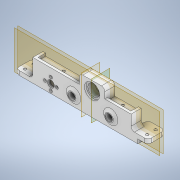
# Autodesk Inventor part: MotorBracketv2
Saved by Autodesk Inventor 2022 (Build 260153000, 153)
## iProperties
Created: 2022-01-31
Part Number: MotorBracketv2
Material: ABS プラスチック
Document SubType Name: Modeling
Designer: shiokaze
Density: 1.06 g/cm^3
Appearance: 滑らか - 白
Mass: 5.74152 g
Surface Area: 41.0545 cm^2
Volume: 5.41653 cm^3
Author: shiokaze
Autodesk Inventor part; units mm, degrees
ref_plane "YZ Plane" through (0, 0, 0) normal (1, 0, 0) x (0, 1, 0)
ref_plane "XZ Plane" through (0, 0, 0) normal (0, 1, 0) x (-1, 0, 0)
ref_plane "XY Plane" through (0, 0, 0) normal (0, 0, 1) x (1, 0, 0)
sketch "スケッチ2" plane through (0, 0, 0) normal (0, 0, 1) x (1, 0, 0)
  line L0 (-46.5, 9.45) -> (31.5, 9.45)
  line L1 (31.5, 9.45) -> (31.5, -9.45)
  line L2 (31.5, -9.45) -> (-46.5, -9.45)
  line L3 (-46.5, -9.45) -> (-46.5, 9.45)
  line L4 (-46.5, 9.45) -> (31.5, -9.45)
  line L5 (31.5, 9.45) -> (-46.5, -9.45)
  line L6 (-46.5, 9.45) -> (-9, 9.45)
  line L7 (-9, 9.45) -> (-9, -6.95)
  line L8 (-9, -6.95) -> (-46.5, -6.95)
  line L9 (-46.5, -6.95) -> (-46.5, 9.45)
  line L10 (31.5, 9.45) -> (6, 9.45)
  line L11 (6, 9.45) -> (6, -4.45)
  line L12 (6, -4.45) -> (31.5, -4.45)
  line L13 (31.5, -4.45) -> (31.5, 9.45)
  line L14 (-36.1825, -6.95) -> (-36.5, -6.95)
  line L15 (-36.5, -6.95) -> (-36.5, 3.75)
  line L16 (-36.5, 3.75) -> (-9, 3.75)
  line L17 (-9, 3.75) -> (-9, -0.3635)
  line L18 (6, -4.45) -> (21.5, -4.45)
  line L19 (21.5, -4.45) -> (21.5, 3.75)
  line L20 (21.5, 3.75) -> (6, 3.75)
  line L21 (6, 3.75) -> (6, -4.45)
  line L22 (31.5, -9.45) -> (25.5, -9.45)
  line L23 (25.5, -9.45) -> (25.5, -6.95)
  line L24 (25.5, -6.95) -> (31.5, -6.95)
  line L25 (31.5, -6.95) -> (31.5, -9.45)
  line L26 (-7.5, 0) -> (0, 0)
  point P0 (-7.5, 0)
  point P1 (6, 3.75)
  point P2 (6, 9.45)
  point P3 (-9, 9.45)
  point P4 (-9, 3.75)
  point P5 (-36.5, -6.95)
  point P6 (25.5, -9.45)
  point P7 (31.5, -6.95)
  point P8 (31.5, -4.45)
  dimension "d0" = 78
  dimension "d1" = 18.9
  dimension "d15" = 37.5
  dimension "d16" = 2.5
  dimension "d17" = 25.5
  dimension "d18" = 6
  dimension "d19" = 2.5
  dimension "d20" = 10
  dimension "d21" = 10
  dimension "d26" = 7.5
  dimension "d188" = 10.7
  dimension "d241" = 5
  constraints: 54 end point, 12 parallel, 7 horizontal, 6 perpendicular, 3 collinear, 2 midpoint, 2 point on line, 1 coincident
  measures "d0" distance of L0.start L0.end
  measures "d1" distance of L0.end L1.end
  measures "d15" distance of L7.end L8.end
  measures "d16" distance between parallel lines of L2 L8
  measures "d17" distance of L12.end L11.end
  measures "d18" distance of L23.end L24.end
  measures "d19" distance of L22.end L23.end
  measures "d20" distance between parallel lines of L1 L19
  measures "d21" distance between parallel lines of L3 L15
  measures "d26" distance of L26.start L26.end
  measures "d188" distance between parallel lines of L16 L8
  measures "d241" distance between parallel lines of L18 L2
extrude "押し出し1" add sketch "スケッチ2" along normal blind 6 contours L0 L11 L5 L4 L7 | L8 L5 L3 | L16 L7 L4 | L4 L7 L5 L8 L15 L16 | L5 L8 L7 L4 L11 L12 L23 L2 | L4 L5 L7 | L20 L5 L11 | L5 L7 L8 | L5 L11 L4 | L1 L24 L23 L4 L12 | L20 L19 L12 L4 L11 L5 | L4 L12 L11
sketch "スケッチ8" plane through (0, 0, 6) normal (0, 0, 1) x (1, 0, 0)
  circle A0 centre (-1.5, 4.0146) radius 3.75 construction
  circle A1 centre (9.5, -3.55) radius 9.6 construction
  circle A2 centre (-12.5, -3.55) radius 9.6 construction
  circle A3 centre (-25.8196, -4.45) radius 3.75 construction
  line L0 (-46.5, -9.45) -> (25.5, -9.45) construction
  circle A4 centre (-12.5, -3.55) radius 10
  circle A5 centre (9.5, -3.55) radius 10
  line L1 (-2.5, -3.55) -> (-0.5, -3.55)
  line L2 (-12.5, -3.55) -> (-1.5, 4.0146) construction
  line L3 (-1.5, 4.0146) -> (9.5, -3.55) construction
  line L4 (-25.8196, -4.45) -> (-12.5, -3.55) construction
  line L5 (-46.5, -9.45) -> (25.5, -9.45) projected
  line L6 (-46.5, -9.45) -> (25.5, -9.45)
  line L7 (25.5, -9.45) -> (25.5, -11.05)
  line L8 (25.5, -11.05) -> (-46.5, -11.05) construction
  line L9 (-46.5, -11.05) -> (-46.5, -9.45)
  line L10 (-46.5, -11.05) -> (25.5, -11.05)
  line L11 (25.5, -11.05) -> (25.5, -13.55)
  line L12 (25.5, -13.55) -> (-46.5, -13.55) construction
  line L13 (-46.5, -13.55) -> (-46.5, -11.05)
  line L14 (25.5, -9.45) -> (25.5, -6.95) projected
  line L15 (6, 9.45) -> (-9, 9.45) projected
  circle A6 centre (-25.8196, -4.45) radius 5
  point P0 (0, 0)
  point P1 (-1.5, 9.45)
  dimension "d123" = 20
  dimension "d124" = 20
  dimension "d29" = 7.5
  dimension "d30" = 19.2
  dimension "d31" = 19.2
  dimension "d32" = 7.5
  dimension "d132" = 2
  dimension "d147" = 1.6
  dimension "d148" = 2.5
  dimension "d164" = 10
  constraints: 24 end point, 7 coincident, 5 centre point, 4 horizontal, 4 parallel, 2 collinear, 2 equal length, 2 horizontal alignment, 2 perpendicular, 2 point on line, 2 tangent, 1 midpoint, 1 vertical alignment, 4 other
  measures "d29" diameter of A0
  measures "d30" diameter of A2
  measures "d31" diameter of A1
  measures "d32" diameter of A3
  measures "d132" distance of L1.start L1.end
  measures "d147" distance of L6.end L7.end
  measures "d148" distance of L10.end L11.end
  measures "d164" diameter of A6
hole "穴1" at (-12.5, -3.55, 6) at (9.5, -3.55, 6) at (-1.5, 4.0146, 6) at (-25.8196, -4.45, 6) direction (0, 0, -1) diameter 0.1 end through all
sketch "スケッチ22" plane through (0, 0, 6) normal (0, 0, 1) x (1, 0, 0)
  circle A0 centre (9.5, -3.55) radius 0.05 projected
  circle A1 centre (-12.5, -3.55) radius 0.05 projected
  circle A2 centre (-25.8196, -4.45) radius 0.05 projected
  point P0 (0, 0)
  constraints: 3 coincident
hole "穴8" at (-12.5, -3.55, 6) at (9.5, -3.55, 6) direction (0, 0, -1) diameter 4 end through all
sketch "スケッチ23" plane through (0, 0, 6) normal (0, 0, 1) x (1, 0, 0)
  circle A0 centre (-1.5, 4.0146) radius 0.05 projected
  point P0 (0, 0)
  constraints: 1 coincident
hole "穴9" at (-1.5, 4.0146, 6) direction (0, 0, -1) diameter 7 end through all
sketch "スケッチ27" plane through (0, 0, 6) normal (0, 0, 1) x (1, 0, 0)
  circle A0 centre (-25.8196, -4.45) radius 0.05 projected
  point P0 (0, 0)
  constraints: 1 coincident
hole "穴10" at (-25.8196, -4.45, 6) direction (0, 0, -1) diameter 10 end through all
sketch "スケッチ28" plane through (0, 0, 6) normal (0, 0, 1) x (1, 0, 0)
  circle A0 centre (-25.8196, -4.45) radius 5 projected
  circle A1 centre (-25.8196, -4.45) radius 2
  point P0 (0, 0)
  point P1 (-25.8196, -9.45)
  dimension "d173" = 4
  constraints: 1 centre point, 1 coincident, 1 vertical alignment
  measures "d173" diameter of A1
extrude "押し出し8" add sketch "スケッチ28" against normal blind 1.5
sketch "スケッチ29" plane through (-25.8196, -4.45, 4.5) normal (0, 0, -1) x (-1, 0, 0)
  circle A0 centre (0, 0) radius 2 projected
  point P0 (-25.8196, 4.45)
  point P1 (-3.5, 0)
  point P2 (0, 3.5)
  point P3 (3.5, 0)
  point P4 (0, -3.5)
  dimension "d176" = 3.5
  dimension "d179" = 360
  constraints: 1 coincident, 1 horizontal alignment, 5 other
  measures "d176" distance of point (0, 0) point (-3.5, 0)
hole "穴11" at (-22.3196, -4.45, 4.5) at (-25.8196, -4.45, 4.5) at (-25.8196, -0.95, 4.5) at (-29.3196, -4.45, 4.5) at (-25.8196, -7.95, 4.5) direction (0, 0, 1) diameter 1.8 end through all
sketch "スケッチ30" plane through (0, 0, 0) normal (0, 0, -1) x (-1, 0, 0)
  circle A0 centre (1.5, 4.0146) radius 3.5 projected
  circle A1 centre (1.5, 4.0146) radius 4.5
  point P0 (0, 0)
  dimension "d189" = 9
  constraints: 1 centre point, 1 coincident
  measures "d189" diameter of A1
extrude "押し出し9" cut sketch "スケッチ30" against normal blind 1
sketch "スケッチ31" plane through (-46.5, -9.45, 6) normal (0, -1, 0) x (1, 0, 0)
  line L0 (49.5, -7.5) -> (40.5, -7.5)
  line L1 (40.5, -7.5) -> (40.5, -2.5)
  line L2 (40.5, -2.5) -> (49.5, -2.5)
  line L3 (49.5, -2.5) -> (49.5, -7.5)
  line L4 (49.5, -6) -> (40.5, -6) projected
  line L5 (49.5, -5) -> (40.5, -5) projected
  line L6 (49.5, -6) -> (40.5, -6) projected
  line L7 (0, 0) -> (72, 0) projected
  line L8 (55, -1.6369) -> (35, -1.6369)
  line L9 (35, -1.6369) -> (35, -10)
  line L10 (35, -10) -> (55, -10)
  line L11 (55, -10) -> (55, -1.6369)
  point P0 (46.5, -6)
  point P1 (45, -10)
  point P2 (45, -7.5)
  dimension "d192" = 5
  dimension "d193" = 7.5
  dimension "d194" = 10
  dimension "d195" = 20
  constraints: 16 end point, 4 midpoint, 4 parallel, 2 horizontal, 2 perpendicular, 1 vertical alignment
  measures "d192" distance between parallel lines of L0 L2
  measures "d193" distance between parallel lines of L0 L7
  measures "d194" distance between parallel lines of L10 L7
  measures "d195" distance of L9.end L10.end
extrude "押し出し10" add sketch "スケッチ31" against normal blind 1.5
sketch "スケッチ32" plane through (-46.5, -9.45, 6) normal (0, -1, 0) x (1, 0, 0)
  line L0 (52.5, -7.5) -> (37.5, -7.5)
  line L1 (52.5, -7.5) -> (37.5, -7.5)
  line L2 (37.5, -7.5) -> (37.5, -2.5)
  line L3 (37.5, -2.5) -> (52.5, -2.5)
  line L4 (52.5, -2.5) -> (52.5, -7.5)
  line L5 (37.5, -7.5) -> (37.5, -6)
  line L6 (41.5, -5) -> (48.5, -5) projected
  line L7 (0, 0) -> (72, 0) projected
  point P0 (45, -2.5)
  point P1 (45, -5)
  dimension "d198" = 5
  dimension "d204" = 15
  dimension "d205" = 2.5
  constraints: 12 end point, 2 midpoint, 2 parallel, 1 collinear, 1 horizontal, 1 perpendicular, 1 vertical alignment
  measures "d198" distance of L1.end L2.end
  measures "d204" distance between parallel lines of L4 L2
  measures "d205" distance between parallel lines of L3 L7
extrude "押し出し11" add sketch "スケッチ32" along normal blind 1.6
sketch "スケッチ33" plane through (-46.5, -9.45, 6) normal (0, 1, 0) x (1, 0, 0)
  line L0 (52.5, 2.5) -> (37.5, 2.5) projected
  line L1 (37.5, 2.5) -> (37.5, 7.5) projected
  line L2 (37.5, 7.5) -> (52.5, 7.5) projected
  line L3 (52.5, 7.5) -> (52.5, 2.5) projected
extrude "押し出し12" add sketch "スケッチ33" along normal up to surface (1.5 mm away)
fillet "フィレット14" radius 2 4 edges at (6, -10.25, -1.5) (6, -10.25, 3.5) (-9, -10.25, -1.5) (-9, -10.25, 3.5)
sketch "スケッチ34" plane through (0, 0, 0) normal (0, 0, -1) x (-1, 0, 0)
  line L0 (-31.5, -4.45) -> (-21.5, -4.45) projected
  line L1 (-31.5, -6.95) -> (-31.5, -4.45) projected
  line L2 (-25.5, -6.95) -> (-31.5, -6.95) projected
  line L3 (-8.5, -9.45) -> (-25.5, -9.45) projected
  line L4 (-25.5, -9.45) -> (-25.5, -6.95) projected
  line L5 (-21.5, -4.45) -> (-21.5, 3.75) projected
  line L6 (36.5, -6.95) -> (46.5, -6.95) projected
  line L7 (36.5, 3.75) -> (36.5, -6.95) projected
  line L8 (46.5, -9.45) -> (25.8196, -9.45) projected
  line L9 (46.5, -6.95) -> (46.5, -9.45) projected
  line L10 (-31.5, -4.45) -> (-21.5, -4.45)
  line L11 (-21.5, -4.45) -> (-21.5, -6.95)
  line L12 (-21.5, -6.95) -> (-31.5, -6.95)
  line L13 (-31.5, -6.95) -> (-31.5, -4.45)
  line L14 (46.5, -9.45) -> (-25.5, -9.45) projected
  line L15 (-21.5, -9.45) -> (-25.5, -9.45)
  line L16 (-25.5, -9.45) -> (-25.5, -6.95)
  line L17 (-25.5, -6.95) -> (-21.5, -6.95)
  line L18 (-21.5, -6.95) -> (-21.5, -9.45)
  line L19 (36.5, -6.95) -> (46.5, -6.95)
  line L20 (46.5, -6.95) -> (46.5, -9.45)
  line L21 (46.5, -9.45) -> (36.5, -9.45)
  line L22 (36.5, -9.45) -> (36.5, -6.95)
  point P0 (0, 0)
  point P1 (36.5, -9.45)
  point P2 (-21.5, -4.45)
  point P3 (-21.5, -9.45)
  constraints: 24 end point, 6 parallel, 3 horizontal, 3 perpendicular, 2 collinear, 2 point on line
extrude "押し出し13" add sketch "スケッチ34" along normal blind 10 from surface at -6
fillet "フィレット15" radius 2 8 edges at (21.5, -6.95, -4) (21.5, -6.95, 0) (-36.5, -8.2, 0) (-36.5, -8.2, -4) (31.5, -5.7, -4) (31.5, -5.7, 6) (-46.5, -8.2, -4) (-46.5, -8.2, 6)
fillet "フィレット16" radius 2 2 edges at (21.5, -4.45, 3) (-36.5, -6.95, 3)
fillet "フィレット17" radius 1.5 5 edges at (8.5, -8.7, -4) (-11.5, -8.7, -4) (-1.5, -7.95, 0) (8.5, -8.7, 0) (-11.5, -8.7, 0)
sketch "スケッチ35" plane through (-36.5, 3.75, 0) normal (0, 1, 0) x (1, 0, 0)
  line L0 (27.5, 0) -> (0, 0) projected
  line L1 (0, 0) -> (0, -6) projected
  line L2 (27.5, -6) -> (0, -6) projected
  line L3 (27.5, 0) -> (27.5, -6) projected
  line L4 (58, 0) -> (42.5, 0) projected
  line L5 (42.5, 0) -> (42.5, -6) projected
  line L6 (58, -6) -> (42.5, -6) projected
  line L7 (58, 0) -> (58, -6) projected
  line L8 (27.5, 0) -> (1.6, 0)
  line L9 (1.6, 0) -> (1.6, -4.5)
  line L10 (1.6, -4.5) -> (27.5, -4.5)
  line L11 (27.5, -4.5) -> (27.5, 0)
  line L12 (42.5, 0) -> (56.4, 0)
  line L13 (56.4, 0) -> (56.4, -4.5)
  line L14 (56.4, -4.5) -> (42.5, -4.5)
  line L15 (42.5, -4.5) -> (42.5, 0)
  point P0 (36.5, 0)
  dimension "d211" = 25.9
  dimension "d212" = 4.5
  dimension "d215" = 13.9
  dimension "d216" = 4.5
  constraints: 16 end point, 4 parallel, 2 horizontal, 2 perpendicular, 1 coincident
  measures "d211" distance of L10.end L9.end
  measures "d212" distance of L8.end L9.end
  measures "d215" distance of L13.end L14.end
  measures "d216" distance of L12.end L13.end
extrude "押し出し14" cut sketch "スケッチ35" against normal blind 1.6 contours L3 L10 L9 L0 | L13 L14 L5 L4
sketch "スケッチ37" plane through (-36.5, 2.15, 0) normal (0, 1, 0) x (1, 0, 0)
  line L0 (27.5, 0) -> (27.5, -6) projected
  line L1 (1.6, 0) -> (27.5, 0) projected
  line L2 (42.5, 0) -> (42.5, -6) projected
  point P0 (36.5, 0)
  point P1 (14.55, -2.25)
  point P2 (49.45, -2.25)
  dimension "d219" = 12.95
  dimension "d220" = 2.25
  dimension "d221" = 6.95
  constraints: 1 horizontal alignment
  measures "d219" distance from line of L0 point (14.55, -2.25)
  measures "d220" distance from line of L1 point (14.55, -2.25)
  measures "d221" distance from line of L2 point (49.45, -2.25)
hole "穴12" at (-21.95, 2.15, 2.25) at (12.95, 2.15, 2.25) direction (0, -1, 0) diameter 1.567 depth 0.1 tip angle 118 thread size "M2x0.4" class "6H" standard "ISO Metric profile"
ref_plane "作業平面3" through (-7.5, -6.95, 4) normal (1, 0, 0) x (0, 0, -1)
ref_plane "作業平面4" through (-1.5, 3.75, 6) normal (-1, 0, 0) x (0, 0, 1)
ref_plane "作業平面5" through (-7, -9.45, 1) normal (0, 0, 1) x (1, 0, 0)
ref_plane "作業平面6" through (0, 0, 3) normal (0, 0, 1) x (1, 0, 0)
sketch "スケッチ40" plane through (23.5, -4.45, -4) normal (0, 1, 0) x (1, 0, 0)
  line L0 (8, -10) -> (5, -10)
  line L1 (5, -10) -> (5, -7.5)
  line L2 (5, -7.5) -> (8, -7.5)
  line L3 (8, -7.5) -> (8, -10)
  line L4 (6, -10) -> (0, -10) projected
  line L5 (8, -2) -> (8, -8) projected
  point P0 (-23.5, -4)
  dimension "d231" = 3
  dimension "d232" = 2.5
  constraints: 8 end point, 2 collinear, 2 parallel, 1 coincident, 1 horizontal, 1 perpendicular
  measures "d231" distance of L1.end L2.end
  measures "d232" distance of L0.end L1.end
hole "穴13" at (28.5, -4.45, 3.5) direction (0, -1, 0) diameter 1.567 depth 0.1 tip angle 118 thread size "M2x0.4" class "6H" standard "ISO Metric profile"
mirror "ミラー2" about plane through (-7, -9.45, 1) normal (0, 0, 1) of "穴13"
fillet "フィレット18" radius 2 2 edges at (6, 9.45, 3) (-9, 9.45, 3)
sketch "スケッチ42" plane through (-44.5, -6.95, -4) normal (0, 1, 0) x (1, 0, 0)
  line L0 (6, -10) -> (0, -10) projected
  line L1 (-2, -2) -> (-2, -8) projected
  line L2 (-2, -10) -> (1, -10)
  line L3 (1, -10) -> (1, -7.5)
  line L4 (1, -7.5) -> (-2, -7.5)
  line L5 (-2, -7.5) -> (-2, -10)
  point P0 (44.5, -4)
  dimension "d242" = 3
  dimension "d243" = 2.5
  constraints: 8 end point, 2 parallel, 1 coincident, 1 collinear, 1 horizontal, 1 perpendicular, 1 point on line
  measures "d242" distance of L4.end L3.end
  measures "d243" distance of L3.end L2.end
hole "穴14" at (-43.5, -6.95, 3.5) direction (0, -1, 0) diameter 1.567 depth 0.1 tip angle 118 thread size "M2x0.4" class "6H" standard "ISO Metric profile"
mirror "ミラー4" about plane through (-7, -9.45, 1) normal (0, 0, 1) of "穴14"
sketch "スケッチ43" plane through (0, 0, 6) normal (0, 0, 1) x (1, 0, 0)
  circle A0 centre (9.5, -3.55) radius 2 projected
  circle A1 centre (9.5, -3.55) radius 2.5
  circle A2 centre (-12.5, -3.55) radius 2 projected
  circle A3 centre (-12.5, -3.55) radius 2.5
  point P0 (0, 0)
  dimension "d251" = 5
  dimension "d252" = 5
  constraints: 2 centre point, 2 coincident
  measures "d251" diameter of A1
  measures "d252" diameter of A3
extrude "押し出し15" add sketch "スケッチ43" along normal blind 1
fillet "フィレット19" radius 2 2 edges at (7, -3.55, 6) (-15, -3.55, 6)
sketch "スケッチ44" plane through (0, 0, 6) normal (0, 0, 1) x (1, 0, 0)
  circle A0 centre (-1.5, 4.0146) radius 4.5 projected
  point P0 (0, 0)
extrude "押し出し16" cut sketch "スケッチ44" against normal blind 1
